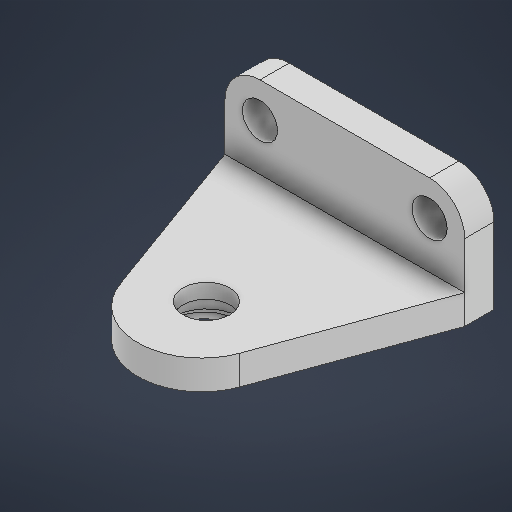
# Autodesk Inventor part: axle support
Saved by Autodesk Inventor 2026 (Build 300175000, 175)
## iProperties
Created: 2025-05-07
Part Number: axle support
Material: Generic
Document SubType Name: Modeling
Designer: Ritul Kumari
Density: 1 g/cm^3
Appearance: Default
Author: Ritul Kumari
Autodesk Inventor part; units mm, degrees
ref_plane "YZ Plane" through (0, 0, 0) normal (1, 0, 0) x (0, 1, 0)
ref_plane "XZ Plane" through (0, 0, 0) normal (0, 1, 0) x (-1, 0, 0)
ref_plane "XY Plane" through (0, 0, 0) normal (0, 0, 1) x (1, 0, 0)
sketch "Sketch1" plane through (0, 0, 0) normal (0, 0, 1) x (1, 0, 0)
  line L0 (-16.3198, 0) -> (-16.3198, 965.2)
  line L1 (-16.3198, 965.2) -> (2066.4802, 965.2)
  line L2 (2066.4802, 965.2) -> (2066.4802, 0)
  line L3 (2066.4802, 0) -> (0, 0)
  line L4 (2066.4802, 0) -> (-16.3198, 0)
  dimension "d0" = 965.2
  dimension "d1" = 2082.8
  constraints: 10 end point, 2 horizontal, 2 perpendicular, 1 vertical
  measures "d0" distance of L0.start L0.end
  measures "d1" distance of L0.end L1.end
extrude "Extrusion1" add sketch "Sketch1" along normal blind 254
fillet "Fillet1" radius 304.8 2 edges at (-16.3198, 965.2, 127) (2066.4802, 965.2, 127)
sketch "Sketch2" plane through (0, 0, 254) normal (0, 0, 1) x (1, 0, 0)
  arc A0 (288.4802, 965.2) -> (-16.3198, 660.4) centre (288.4802, 660.4) ccw projected
  circle A1 centre (288.4802, 660.4) radius 152.4
  point P0 (0, 0)
  dimension "d5" = 304.8
  constraints: 1 centre point, 1 coincident
  measures "d5" diameter of A1
hole "Hole1" at (288.4802, 660.4, 254) direction (0, 0, -1) diameter 304.8 end through all
sketch "Sketch3" plane through (0, 0, 254) normal (0, 0, 1) x (1, 0, 0)
  arc A0 (2066.4802, 660.4) -> (1761.6802, 965.2) centre (1761.6802, 660.4) ccw projected
  circle A1 centre (1761.6802, 660.4) radius 152.4
  point P0 (0, 0)
  dimension "d13" = 304.8
  constraints: 1 centre point, 1 coincident
  measures "d13" diameter of A1
hole "Hole2" at (1761.6802, 660.4, 254) direction (0, 0, -1) diameter 304.8 end through all
sketch "Sketch4" plane through (0, 0, 0) normal (0, 1, 0) x (-1, 0, 0)
  line L0 (16.3198, 254) -> (-2066.4802, 254) projected
  line L1 (16.3198, 254) -> (-1025.0802, 254)
  line L2 (-1025.0802, 254) -> (-1025.0802, 1473.2)
  line L3 (16.3198, 254) -> (-504.9189, 1686.0916)
  line L4 (16.3198, 254) -> (1540.3198, 254) construction
  line L5 (-2066.4802, 254) -> (-1545.2415, 1686.0916)
  line L6 (-2066.4802, 254) -> (-542.4802, 254) construction
  arc A0 (-504.9189, 1686.0916) -> (-1545.2415, 1686.0916) centre (-1025.0802, 1496.7683) ccw
  point P0 (0, 0)
  dimension "d21" = 1219.2
  dimension "d22" = 1524
  dimension "d23" = 110
  dimension "d24" = 1524
  dimension "d25" = 70
  constraints: 12 end point, 2 equal length, 2 horizontal, 2 point on circle, 1 centre point, 1 midpoint, 1 perpendicular, 1 tangent
  measures "d21" distance of L1.end L2.end
  measures "d22" distance of L0.start L3.end
  measures "d23" angle of L4 L3
  measures "d24" distance of L0.end L5.end
  measures "d25" angle of L6 L5
extrude "Extrusion2" add sketch "Sketch4" along normal blind 254
sketch "Sketch5" plane through (0, 0, 0) normal (0, 0, -1) x (-1, 0, 0)
  point P0 (0, 0)
  point P1 (-179.0917, -175.9118)
  point P2 (-179.0917, -175.9118)
  constraints: 1 coincident
sketch "Sketch6" plane through (0, 0, 0) normal (0, 1, 0) x (-1, 0, 0)
  line L0 (-2066.4802, 0) -> (-2066.4802, 254) projected
  line L1 (-2066.4802, 0) -> (-1025.0802, 0)
  line L2 (-1609.2802, 0) -> (-1914.0802, 0) projected
  line L3 (-1025.0802, 0) -> (-1025.0802, 1473.2)
  circle A0 centre (-1025.0802, 1473.2) radius 203.2
  circle A1 centre (-1025.0802, 1473.2) radius 279.4
  circle A2 centre (-1025.0802, 1473.2) radius 431.8
  point P0 (0, 0)
  dimension "d28" = 1041.4
  dimension "d29" = 1473.2
  dimension "d30" = 406.4
  dimension "d31" = 558.8
  dimension "d32" = 863.6
  constraints: 4 end point, 3 centre point, 3 coincident, 1 collinear, 1 perpendicular
  measures "d28" distance of L0.start L1.end
  measures "d29" distance of L1.end L3.end
  measures "d30" diameter of A0
  measures "d31" diameter of A1
  measures "d32" diameter of A2
extrude "Extrusion3" add sketch "Sketch6" against normal blind 50.8 contours A2
sketch "Sketch7" plane through (0, 0, 0) normal (0, 1, 0) x (-1, 0, 0)
  circle A0 centre (-1025.0802, 1473.2) radius 279.4 projected
  circle A1 centre (-1025.0802, 1473.2) radius 203.2
  point P0 (0, 0)
  point P1 (-1010.2805, 1441.3983)
  dimension "d35" = 406.4
  constraints: 1 centre point, 1 coincident
  measures "d35" diameter of A1
hole "Hole3" at (1010.2805, 0, 1441.3983) direction (0, 1, 0) diameter 406.4 end through all counterbore diameter 558.8 counterbore depth 127
body "Solid1"
